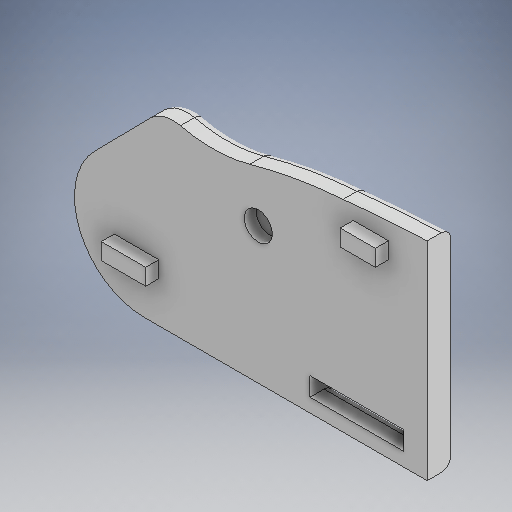
# Autodesk Inventor part: Part7
Saved by Autodesk Inventor 2025.2 (Build 292293000, 293)
## iProperties
Created: 2025-02-14
Part Number: Part7
Material: Generic
Document SubType Name: Modeling
Designer: Alex
Density: 1 g/cm^3
Appearance: Default
Author: Alex
Autodesk Inventor part; units mm, degrees
ref_plane "YZ Plane" through (0, 0, 0) normal (1, 0, 0) x (0, 1, 0)
ref_plane "XZ Plane" through (0, 0, 0) normal (0, 1, 0) x (-1, 0, 0)
ref_plane "XY Plane" through (0, 0, 0) normal (0, 0, 1) x (1, 0, 0)
sketch "Sketch1" plane through (0, 0, 0) normal (0, 0, 1) x (1, 0, 0)
  line L0 (23.5502, -2.4906) -> (23.5502, 41.9756)
  line L1 (23.5502, 41.9756) -> (-24.3513, 41.9756)
  arc A0 (-24.3513, 41.9756) -> (-51.4155, 40.4994) centre (-24.3513, -206.8647) ccw
  arc A1 (-51.4155, 40.4994) -> (-53.2937, 36.872) centre (-51.1487, 38.0613) ccw
  arc A2 (-52.4631, 18.3802) -> (-53.2937, 36.872) centre (-71.4744, 26.7908) ccw
  arc A3 (-52.4631, 18.3802) -> (-51.5486, 16.9756) centre (-51.5486, 17.9756) ccw
  line L2 (-51.5486, 16.9756) -> (-49.1487, 16.9756)
  arc A4 (-49.1487, 16.9756) -> (-41.1487, 24.9756) centre (-49.1487, 24.9756) ccw
  line L3 (-41.1487, 24.9756) -> (-41.1487, 25.9756)
  arc A5 (-33.1487, 33.9756) -> (-41.1487, 25.9756) centre (-33.1487, 25.9756) ccw
  line L4 (-33.1487, 33.9756) -> (7.8511, 33.9756)
  arc A6 (15.8511, 25.9756) -> (7.8511, 33.9756) centre (7.8511, 25.9756) ccw
  line L5 (15.8511, 25.9756) -> (15.8511, 15.4748)
  arc A7 (7.8511, 7.4748) -> (15.8511, 15.4748) centre (7.8511, 15.4748) ccw
  arc A8 (-85.7245, 35.8004) -> (-77.2609, 7.4748) centre (-71.1949, 24.7145) ccw
  arc A9 (-85.7245, 35.8004) -> (-86.0748, 36.7885) centre (-86.2221, 36.1801) ccw
  arc A10 (-86.0748, 36.7885) -> (-92.5086, 34.981) centre (-87.6817, 30.154) ccw
  line L6 (-92.5086, 34.981) -> (-126.1935, 1.2961)
  arc A11 (-126.7239, 0.8028) -> (-126.1935, 1.2961) centre (-133.2646, 8.3671) ccw
  arc A12 (-51.4155, 40.4994) -> (-53.2937, 36.872) centre (-51.1487, 38.0613) ccw
  arc A13 (-51.4155, 40.4994) -> (-71.2834, 37.0539) centre (-44.4816, -58.4873) ccw
  arc A14 (-86.0748, 36.7885) -> (-71.2834, 37.0539) centre (-79.1869, 65.2278) ccw
  line L7 (7.8511, 7.4748) -> (-77.2609, 7.4748)
  line L8 (-126.7239, 0.8028) -> (-130.5327, -2.4906)
  line L9 (-130.5327, -2.4906) -> (23.5502, -2.4906)
  point P0 (0, 0)
  point P1 (-126.1489, 0.9748)
  dimension "d0" = 8
  dimension "d1" = 248.8403
  dimension "d2" = 99.2292
  dimension "d3" = 2.4527
  dimension "d4" = 2.4527
  dimension "d5" = 1
  dimension "d6" = 18.2758
  dimension "d7" = 20.7887
  dimension "d8" = 29.2615
  dimension "d9" = 0.626
  dimension "d10" = 6.8264
  dimension "d11" = 10
  dimension "d12" = 135
  dimension "d13" = 139.151
  dimension "d14" = 34.5008
  dimension "d15" = 8
  dimension "d16" = 25
  dimension "d17" = 44.4661
  dimension "d18" = 7.6992
  dimension "d19" = 64.699
  dimension "d20" = 41.9756
  dimension "d21" = 23.5502
  dimension "d22" = 90.1488
  dimension "d23" = 83.4934
  dimension "d24" = 47.9015
  dimension "d25" = 100.4628
  dimension "d26" = 68.0318
  dimension "d27" = 75.0988
  dimension "d28" = 17.261
  dimension "d29" = 94.7452
  dimension "d30" = 41.0008
  dimension "d31" = 149.6992
  constraints: 30 point on circle, 20 end point, 20 tangent, 15 centre point, 6 parallel, 3 equal radius, 1 horizontal, 1 vertical
  measures "d0" radius of A6
  measures "d1" radius of A0
  measures "d2" radius of A13
  measures "d3" radius of A12
  measures "d4" radius of A1
  measures "d5" radius of A3
  measures "d6" radius of A8
  measures "d7" radius of A2
  measures "d8" radius of A14
  measures "d9" radius of A9
  measures "d10" radius of A10
  measures "d11" radius of A11
  measures "d12" angle of L1 L6
  measures "d13" angle of L1 L8
  measures "d14" distance between parallel lines of L1 L7
  measures "d15" distance between parallel lines of L1 L4
  measures "d16" distance between parallel lines of L1 L2
  measures "d17" distance between parallel lines of L1 L9
  measures "d18" distance between parallel lines of L0 L5
  measures "d19" distance between parallel lines of L0 L3
  measures "d20" distance from line of point (0, 0) L1
  measures "d21" distance from line of point (0, 0) L0
  measures "d22" distance from line of point (0, 0) L6
  measures "d23" distance from line of point (0, 0) L8
  measures "d24" distance from line of L1.end L0
  measures "d25" distance from line of A13.centre L1
  measures "d26" distance from line of A13.centre L0
  measures "d27" distance from line of A3.centre L0
  measures "d28" distance from line of A8.centre L1
  measures "d29" distance from line of A8.centre L0
  measures "d30" distance from line of point (-126.149, 0.975) L1
  measures "d31" distance from line of point (-126.149, 0.975) L0
sketch "Sketch2" plane through (0, 0, 0) normal (0, 0, 1) x (1, 0, 0)
  line L0 (-33.4498, 41.8092) -> (-33.4498, -2.4906)
  line L1 (23.5502, -2.4906) -> (23.5502, 41.9756) construction
  line L2 (23.5502, 41.9756) -> (-24.3513, 41.9756) construction
  arc A0 (-24.3513, 41.9756) -> (-51.4155, 40.4994) centre (-24.3513, -206.8647) ccw projected
  arc A1 (-51.4155, 40.4994) -> (-71.2834, 37.0539) centre (-44.4816, -58.4873) ccw projected
  arc A2 (-86.0748, 36.7885) -> (-71.2834, 37.0539) centre (-79.1869, 65.2278) ccw projected
  arc A3 (-86.0748, 36.7885) -> (-92.5086, 34.981) centre (-87.6817, 30.154) ccw projected
  line L3 (-92.5086, 34.981) -> (-126.1935, 1.2961) construction
  line L4 (-126.7239, 0.8028) -> (-130.5327, -2.4906) construction
  line L5 (-130.5327, -2.4906) -> (23.5502, -2.4906) construction
  arc A4 (7.8511, 7.4748) -> (15.8511, 15.4748) centre (7.8511, 15.4748) ccw construction
  line L6 (15.8511, 25.9756) -> (15.8511, 15.4748) construction
  arc A5 (15.8511, 25.9756) -> (7.8511, 33.9756) centre (7.8511, 25.9756) ccw construction
  line L7 (-33.1487, 33.9756) -> (7.8511, 33.9756) construction
  arc A6 (-33.1487, 33.9756) -> (-41.1487, 25.9756) centre (-33.1487, 25.9756) ccw construction
  arc A7 (-49.1487, 16.9756) -> (-41.1487, 24.9756) centre (-49.1487, 24.9756) ccw construction
  arc A8 (-52.4631, 18.3802) -> (-51.5486, 16.9756) centre (-51.5486, 17.9756) ccw construction
  arc A9 (-52.4631, 18.3802) -> (-53.2937, 36.872) centre (-71.4744, 26.7908) ccw construction
  arc A10 (-51.4155, 40.4994) -> (-53.2937, 36.872) centre (-51.1487, 38.0613) ccw construction
  arc A11 (-85.7245, 35.8004) -> (-77.2609, 7.4748) centre (-71.1949, 24.7145) ccw construction
  arc A12 (-85.7245, 35.8004) -> (-86.0748, 36.7885) centre (-86.2221, 36.1801) ccw construction
  line L8 (7.8511, 7.4748) -> (-77.2609, 7.4748) construction
  line L9 (-41.4498, 37.9652) -> (-49.4498, 37.9652) construction
  line L10 (-49.4498, 37.9652) -> (-49.4498, 33.9652) construction
  line L11 (-49.4498, 33.9652) -> (-41.4498, 33.9652) construction
  line L12 (-41.4498, 33.9652) -> (-41.4498, 37.9652) construction
  line L13 (-49.1998, 37.7152) -> (-41.6998, 37.7152)
  line L14 (-41.6998, 37.7152) -> (-41.6998, 34.2152)
  line L15 (-41.6998, 34.2152) -> (-49.1998, 34.2152)
  line L16 (-49.1998, 34.2152) -> (-49.1998, 37.7152)
  line L17 (-90.4498, 9.9652) -> (-100.4498, 9.9652) construction
  line L18 (-100.4498, 9.9652) -> (-100.4498, 5.9652) construction
  line L19 (-100.4498, 5.9652) -> (-90.4498, 5.9652) construction
  line L20 (-90.4498, 5.9652) -> (-90.4498, 9.9652) construction
  line L21 (-100.1998, 9.7152) -> (-90.6998, 9.7152)
  line L22 (-90.6998, 9.7152) -> (-90.6998, 6.2152)
  line L23 (-90.6998, 6.2152) -> (-100.1998, 6.2152)
  line L24 (-100.1998, 6.2152) -> (-100.1998, 9.7152)
  line L25 (-38.4498, 4.4352) -> (-58.4498, 4.4352)
  line L26 (-58.4498, 4.4352) -> (-58.4498, 0.4352)
  line L27 (-58.4498, 0.4352) -> (-38.4498, 0.4352)
  line L28 (-38.4498, 0.4352) -> (-38.4498, 4.4352)
  line L29 (-33.4498, -2.4906) -> (-130.5327, -2.4906) construction
  line L30 (-93.7668, 2.4352) -> (-93.7668, -6.5217) construction
  circle A13 centre (-93.7685, 12.4352) radius 14.9258 construction
  line L31 (-92.5086, 34.981) -> (-104.4008, 22.9105)
  arc A14 (-104.4008, 22.9105) -> (-93.7668, -2.4906) centre (-93.7685, 12.4352) ccw
  line L32 (-93.7668, -2.4906) -> (-33.4498, -2.4906)
  circle A15 centre (-69.4668, 26.5732) radius 3
  point P0 (0, 0)
  point P1 (-45.4498, 33.9652)
  dimension "d33" = 57
  dimension "d34" = 8
  dimension "d35" = 4
  dimension "d36" = 8
  dimension "d37" = 3.844
  dimension "d38" = 0.25
  dimension "d39" = 41
  dimension "d40" = 24
  dimension "d41" = 10
  dimension "d42" = 4
  dimension "d43" = 0.25
  dimension "d44" = 29.53
  dimension "d45" = 9
  dimension "d46" = 20
  dimension "d47" = 4
  dimension "d48" = 2.47
  dimension "d52" = 3.317
  dimension "d53" = 4.137
  dimension "d59" = 20.017
  dimension "d60" = 7.392
  dimension "d61" = 6
  constraints: 50 end point, 10 parallel, 5 perpendicular, 5 point on circle, 3 centre point, 3 horizontal, 3 point on line, 2 collinear, 2 tangent, 2 vertical, 1 coincident, 1 concentric, 1 midpoint, 6 other
  measures "d33" distance between parallel lines of L0 L1
  measures "d34" distance between parallel lines of L12 L0
  measures "d35" distance from line of point (-45.45, 33.965) L9
  measures "d36" distance between parallel lines of L10 L12
  measures "d37" distance from line of L9 L0.start
  measures "d38" distance between parallel lines of L9 L13
  measures "d39" distance between parallel lines of L20 L10
  measures "d40" distance between parallel lines of L17 L11
  measures "d41" distance of L18.end L19.end
  measures "d42" distance of L17.end L18.end
  measures "d43" distance between parallel lines of L17 L21
  measures "d44" distance between parallel lines of L25 L11
  measures "d45" distance between parallel lines of L26 L10
  measures "d46" distance of L26.end L27.end
  measures "d47" distance of L27.end L25.start
  measures "d48" distance from line of L17 point (-93.768, 12.435)
  measures "d52" distance between parallel lines of L30 L20
  measures "d53" distance of point (-93.768, 12.435) L17.start
  measures "d59" distance from line of A15.centre L10
  measures "d60" distance from line of A15.centre L11
  measures "d61" diameter of A15
extrude "Extrusion1" add sketch "Sketch2" along normal blind 5 contours L0 L32 A14 L31 A3 A2 A1 A0 | L13 L14 L15 L16 | L21 L22 L23 L24 | A15
extrude "Extrusion2" add sketch "Sketch2" along normal blind 7.8 contours L13 L14 L15 L16 | L21 L22 L23 L24
sketch "Sketch3" plane through (0, 0, 5) normal (0, 0, 1) x (1, 0, 0)
  circle A0 centre (-69.4668, 26.5732) radius 3 projected
  point P0 (0, 0)
extrude "Extrusion3" cut sketch "Sketch3" against normal blind 2.5
fillet "Fillet1" radius 2 1 edges at (-48.4498, 0.4352, 0)
fillet "Fillet2" radius 2 7 edges at (-42.4445, 41.3169, 0) (-78.662, 35.971, 0) (-89.528, 36.7259, 0) (-61.4372, 39.2826, 0) (-107.5364, 6.6713, 0) (-63.6083, -2.4906, 0) (-98.4547, 28.9457, 0)
body "Solid1"
